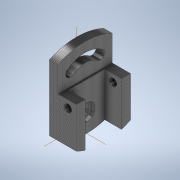
# Autodesk Inventor part: swivel plate
Saved by Autodesk Inventor 2021.1 (Build 251245000, 245)
## iProperties
Created: 2021-02-18
Part Number: swivel plate
Material: Generic
Document SubType Name: Modeling
Designer: Vamshi
Density: 1 g/cm^3
Appearance: Engine Turned
Author: Vamshi
Autodesk Inventor part; units mm, degrees
ref_plane "YZ Plane" through (0, 0, 0) normal (1, 0, 0) x (0, 1, 0)
ref_plane "XZ Plane" through (0, 0, 0) normal (0, 1, 0) x (-1, 0, 0)
ref_plane "XY Plane" through (0, 0, 0) normal (0, 0, 1) x (1, 0, 0)
sketch "Sketch1" plane through (0, 0, 0) normal (1, 0, 0) x (0, 1, 0)
  arc A0 (11.5026, 48.5) -> (11.5026, -48.5) centre (108, 0) ccw
  arc A1 (130.1868, -48.5) -> (130.1868, 48.5) centre (26.826, 0) ccw
  line L0 (11.5026, 48.5) -> (130.1868, 48.5)
  line L1 (130.1868, -48.5) -> (11.5026, -48.5)
  line L2 (0, 0) -> (141, 0)
  arc A2 (107, -27) -> (107, 27) centre (71, 0) ccw construction
  arc A3 (113.4, -31.8) -> (113.4, 31.8) centre (71, 0) ccw
  arc A4 (100.6, -22.2) -> (100.6, 22.2) centre (71, 0) ccw
  arc A5 (100.6, -22.2) -> (113.4, -31.8) centre (107, -27) ccw
  arc A6 (113.4, 31.8) -> (100.6, 22.2) centre (107, 27) ccw
  dimension "d0" = 108
  dimension "d2" = 141
  dimension "d3" = 97
  dimension "d4" = 54
  dimension "d5" = 8
  dimension "d6" = 45
  constraints: 17 point on circle, 7 centre point, 6 end point, 4 tangent, 3 vertical alignment, 1 coincident, 1 horizontal, 1 parallel, 1 point on line
  measures "d0" radius of A0
  measures "d2" distance of L2.start L2.end
  measures "d3" distance between parallel lines of L1 L0
  measures "d4" distance of A2.start A2.end
  measures "d5" radius of A5
  measures "d6" radius of A2
extrude "Extrusion1" add sketch "Sketch1" along normal blind 48 contours L0 A1 L2 A3 A6 A4 A0 | L2 A4 A5 A3 A1 L1 A0
sketch "Sketch2" plane through (48, 0, 0) normal (1, 0, 0) x (0, 0, -1)
  line L0 (-88.6528, 151.7053) -> (89.775, 151.7053)
  line L1 (89.775, 151.7053) -> (89.775, 84)
  line L2 (89.775, 84) -> (-88.6528, 84)
  line L3 (-88.6528, 84) -> (-88.6528, 151.7053)
  point P0 (0, 0)
  dimension "d9" = 84
  constraints: 8 end point, 2 parallel, 1 horizontal, 1 perpendicular
  measures "d9" distance from line of L2 point (0, 0)
extrude "Extrusion2" cut sketch "Sketch2" against normal blind 33
sketch "Sketch3" plane through (48, 0, 0) normal (1, 0, 0) x (0, 0, -1)
  line L0 (48.5, 84) -> (-48.5, 84) projected
  line L1 (-32.5, 84) -> (32.5, 84)
  line L2 (32.5, 84) -> (32.5, -13.4662)
  line L3 (32.5, -13.4662) -> (-32.5, -13.4662)
  line L4 (-32.5, -13.4662) -> (-32.5, 84)
  line L5 (-48.5, 84) -> (-48.5, 11.5026) projected
  line L6 (48.5, 11.5026) -> (48.5, 84) projected
  point P0 (0, 0)
  dimension "d12" = 16
  dimension "d13" = 16
  constraints: 8 end point, 2 parallel, 1 horizontal, 1 perpendicular, 1 point on line
  measures "d12" distance between parallel lines of L5 L4
  measures "d13" distance between parallel lines of L6 L2
extrude "Extrusion3" cut sketch "Sketch3" against normal blind 30
sketch "Sketch4" plane through (0, 11.5026, 48.5) normal (0, 0, 1) x (1, 0, 0)
  circle A0 centre (33, 59.4974) radius 6.5
  line L0 (48, 72.4974) -> (15, 72.4974) projected
  line L1 (48, 72.4974) -> (48, 0) projected
  point P0 (0, -11.5026)
  dimension "d16" = 13
  dimension "d17" = 13
  dimension "d18" = 15
  constraints: 1 centre point
  measures "d16" diameter of A0
  measures "d17" distance from line of L0 A0.centre
  measures "d18" distance from line of A0.centre L1
extrude "Extrusion4" cut sketch "Sketch4" against normal through all
sketch "Sketch5" plane through (18, 0, 0) normal (1, 0, 0) x (0, 0, -1)
  point P0 (0, 0)
  point P1 (0, 33)
  dimension "d21" = 33
  measures "d21" distance of point (0, 0) point (0, 33)
hole "Hole1" at (18, 33, 0) direction (-1, 0, 0) diameter 21 end through all counterbore diameter 30 counterbore depth 6
body "Solid1"
